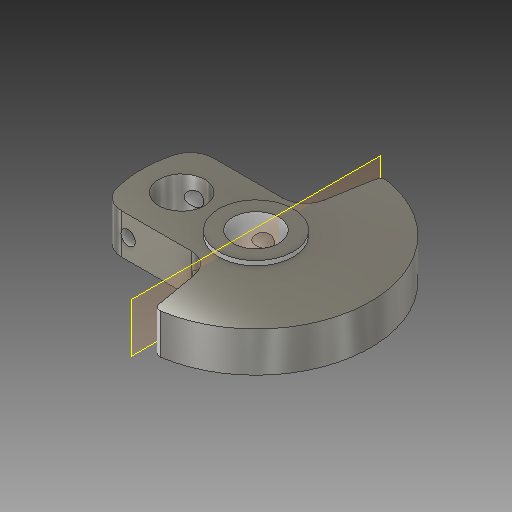
# Autodesk Inventor part: reverse gear crankshaft counter weight 2
Saved by Autodesk Inventor 2017 (Build 210142000, 142)
## iProperties
Created: 2018-11-01
Part Number: reverse gear crankshaft counter weight 2
Material: Generic
Document SubType Name: Modeling
Designer: User
Density: 1 g/cm^3
Appearance: Default
Author: User
Autodesk Inventor part; units mm, degrees
ref_plane "XZ Plane" through (0, 0, 0) normal (0, 1, 0) x (-1, 0, 0)
sketch "Sketch1" plane through (0, 0, 0) normal (0, 1, 0) x (-1, 0, 0)
  line L0 (20, 0) -> (20, -8) construction
  line L1 (20, -8) -> (20, 8)
  line L2 (20, 8) -> (0, 8)
  line L3 (20, -8) -> (0, -8)
  line L4 (0, -8) -> (-2.0965, -19.8898)
  line L5 (0, 8) -> (-2.0965, 19.8898)
  arc A0 (-2.0965, 19.8898) -> (-2.0965, -19.8898) centre (0, 0) ccw construction
  arc A1 (18.3303, -8) -> (18.3303, 8) centre (0, 0) ccw construction
  arc A2 (-2.0965, 19.8898) -> (-2.0965, -19.8898) centre (0, 0) ccw
  arc A3 (18.3303, -8) -> (18.3303, 8) centre (0, 0) ccw
  circle A4 centre (0, 0) radius 20 construction
  circle A5 centre (13, 0) radius 4
  circle A6 centre (0, 0) radius 4
  circle A7 centre (0, 0) radius 6.5
  dimension "d1" = 8
  dimension "d2" = 16
  dimension "d3" = 20
  dimension "d4" = 20
  dimension "d5" = 100
  dimension "d6" = 100
  dimension "d7" = 40
  dimension "d8" = 20
  dimension "d10" = 8
  dimension "d14" = 8
  dimension "d15" = 13
  dimension "d16" = 13
  dimension "d21" = 7
  constraints: 12 end point, 9 point on circle, 8 centre point, 5 coincident, 2 horizontal, 2 point on line, 2 tangent, 2 vertical
  measures "d1" distance of L0.start L0.end
  measures "d2" distance of L0.end L1.end
  measures "d3" distance of L1.end L2.end
  measures "d4" distance of L0.end L3.end
  measures "d5" angle of L3 L4
  measures "d6" angle of L2 L5
  measures "d7" diameter of A4
  measures "d8" radius of A0
  measures "d10" diameter of A5
  measures "d14" diameter of A6
  measures "d15" diameter of A7
  measures "d16" distance of A7.centre A5.centre
  measures "d21" distance from line of A5.centre L0
extrude "Extrusion4" add sketch "Sketch1" along normal blind 7 contours A3 L3 L4 A2 L5 L2
extrude "Extrusion5" add sketch "Sketch1" along normal blind 7.8 contours A7
fillet "Fillet1" radius 4 1 edges at (-18.3303, 3.5, 8)
fillet "Fillet2" radius 4 1 edges at (-18.3303, 3.5, -8)
fillet "Fillet3" radius 4 2 edges at (0, 3.5, -8) (0, 3.5, 8)
fillet "Fillet4" radius 1 2 edges at (2.0965, 3.5, 19.8898) (2.0965, 3.5, -19.8898)
ref_plane "Work Plane1" through (0, 0, 0) normal (0, -1, 0) x (1, 0, 0)
sketch "Sketch3" plane through (-15.4919, 0, 8) normal (0, 0, 1) x (1, 0, 0)
  line L0 (6.4919, 0) -> (-1.5081, 0) projected
  line L1 (0, 7) -> (12.1355, 7) projected
  line L2 (-3.873, 7) -> (0, 7) projected
  line L3 (0, 0) -> (-3.873, 0) projected
  line L4 (-1.5081, 7) -> (6.4919, 7) projected
  line L5 (6.4919, 0) -> (-1.5081, 0) projected
  line L6 (19.4919, 0) -> (11.4919, 0) projected
  line L7 (6.4919, 0) -> (-1.5081, 0) projected
  line L8 (18.5607, 0) -> (17.4225, 0) projected
  line L9 (18.5607, 0) -> (18.5607, 0) projected
  line L10 (17.4225, 0) -> (18.5607, 0) projected
  line L11 (16.0748, 0) -> (17.4225, 0) projected
  line L12 (12.1355, 0) -> (16.0748, 0) projected
  line L13 (0, 0) -> (12.1355, 0) projected
  line L14 (-3.873, 0) -> (0, 0) projected
  line L15 (-3.873, 0) -> (-3.873, 0) projected
  line L16 (0, 0) -> (-3.873, 0) projected
  line L17 (12.1355, 0) -> (0, 0) projected
  line L18 (16.0748, 0) -> (12.1355, 0) projected
  line L19 (17.4225, 0) -> (16.0748, 0) projected
  circle A0 centre (1.1355, 3.4977) radius 1.25
  line L20 (12.1355, 7) -> (12.1355, 0) projected
  point P0 (15.4919, 0)
  dimension "d33" = 2.5
  dimension "d34" = 11
  dimension "d35" = 3.4977
  constraints: 1 centre point
  measures "d33" diameter of A0
  measures "d34" distance from line of L20 A0.centre
  measures "d35" distance from line of A0.centre L0
extrude "Extrusion6" cut sketch "Sketch3" against normal through all
ref_plane "Work Plane2" through (0, 0, 11.5) normal (0, 0, 1) x (1, 0, 0)
sketch "Sketch5" plane through (0, 0, 11.5) normal (0, 0, 1) x (1, 0, 0)
  line L0 (0.5828, 0) -> (0.5828, 7) projected
  line L1 (0.5828, 0) -> (1.9305, 0) construction
  line L2 (0.5828, 0) -> (-4.4172, 0) construction
  line L3 (-4.4172, 0) -> (-4.4172, 7) construction
  line L4 (-4.4172, 7) -> (0.5828, 7) construction
  line L5 (-4.4172, 0) -> (-4.4172, 3.5) construction
  line L6 (-4.4172, 7) -> (-1.9172, 7) construction
  circle A0 centre (-1.9172, 3.5) radius 1.25
  point P0 (0, 0)
  dimension "d45" = 5
  dimension "d46" = 7
  dimension "d47" = 5
  dimension "d48" = 3.5
  dimension "d50" = 2.5
  constraints: 10 end point, 2 midpoint, 1 centre point, 1 horizontal, 1 perpendicular, 1 vertical
  measures "d45" distance of L0.start L2.end
  measures "d46" distance of L2.end L3.end
  measures "d47" distance of L3.end L0.end
  measures "d48" distance of L2.end L5.end
  measures "d50" diameter of A0
extrude "Extrusion7" cut sketch "Sketch5" against normal through all
body "Solid3"
